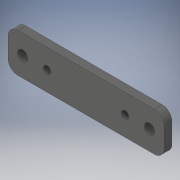
# Autodesk Inventor part: Parts_PCB_BatteryProbePCB
Saved by Autodesk Inventor 2019.1 (Build 231200000, 200)
## iProperties
Created: 2018-08-27
Part Number: Parts_PCB_BatteryProbePCB
Material: ガラス繊維バット
Document SubType Name: Modeling
Designer: sktom
Density: 0.032 g/cm^3
Appearance: 灰色
Author: sktom
Autodesk Inventor part; units mm, degrees
ref_plane "YZ Plane" through (0, 0, 0) normal (1, 0, 0) x (0, 1, 0)
ref_plane "XZ Plane" through (0, 0, 0) normal (0, 1, 0) x (-1, 0, 0)
ref_plane "XY Plane" through (0, 0, 0) normal (0, 0, 1) x (1, 0, 0)
sketch "スケッチ1" plane through (0, 0, 0) normal (0, 0, 1) x (1, 0, 0)
  line L0 (16, -4) -> (-16, -4)
  line L1 (-16, -4) -> (-16, 4)
  line L2 (-16, 4) -> (16, 4)
  line L3 (16, 4) -> (16, -4)
  line L4 (16, -4) -> (-16, 4) construction
  line L5 (-16, -4) -> (16, 4) construction
  circle A0 centre (8, 0) radius 0.75
  circle A1 centre (13, 0) radius 1.05
  circle A2 centre (-8, 0) radius 0.75
  circle A3 centre (-13, 0) radius 1.05
  point P0 (0, 0)
  point P1 (0, 0)
  point P2 (0, 0)
  dimension "d0" = 8
  dimension "d1" = 8
  dimension "d2" = 8
  dimension "d3" = 1.5
  dimension "d4" = 2.1
  dimension "d5" = 13
  dimension "d6" = 3
  dimension "d7" = 13
  constraints: 12 end point, 4 centre point, 4 horizontal alignment, 4 midpoint, 2 equal radius, 2 parallel, 1 horizontal, 1 perpendicular
  measures "d0" distance of L2.end L0.start
  measures "d1" distance of point (0, 0) A0.centre
  measures "d2" distance of point (0, 0) A2.centre
  measures "d3" diameter of A2
  measures "d4" diameter of A1
  measures "d5" distance of point (0, 0) A1.centre
  measures "d6" distance from line of A1.centre L3
  measures "d7" distance of A3.centre point (0, 0)
extrude "押し出し1" add sketch "スケッチ1" along normal blind 1.6
fillet "フィレット1" radius 2 4 edges at (-16, 4, 0.8) (16, 4, 0.8) (16, -4, 0.8) (-16, -4, 0.8)
